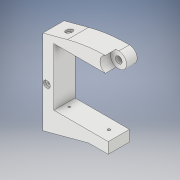
# Autodesk Inventor part: Riser Base
Saved by Autodesk Inventor 2017 SP1 (Build 210196100, 196)
## iProperties
Created: 2017-07-19
Part Number: Riser Base
Material: ABS Plastic
Document SubType Name: Modeling
Designer: zallen
Density: 1.06 g/cm^3
Appearance: CR White
Author: zallen
Autodesk Inventor part; units mm, degrees
ref_plane "YZ Plane" through (0, 0, 0) normal (1, 0, 0) x (0, 1, 0)
ref_plane "XZ Plane" through (0, 0, 0) normal (0, 1, 0) x (-1, 0, 0)
ref_plane "XY Plane" through (0, 0, 0) normal (0, 0, 1) x (1, 0, 0)
sketch "Sketch1" plane through (0, 0, 0) normal (0, 0, 1) x (1, 0, 0)
  line L0 (0, 0) -> (160, 0) construction
  line L1 (160, 0) -> (118.589, -154.5481) construction
  line L2 (0, 0) -> (41.411, -154.5481) construction
  line L3 (41.411, -154.5481) -> (118.589, -154.5481)
  circle A0 centre (235.8871, -103.156) radius 80 construction
  line L4 (160, 0) -> (256.5926, -25.8819)
  line L5 (118.589, -154.5481) -> (215.1815, -180.43)
  arc A1 (215.1815, -180.43) -> (256.5926, -25.8819) centre (235.8871, -103.156) ccw
  circle A2 centre (-75.8871, -103.156) radius 80 construction
  line L6 (0, 0) -> (-96.5926, -25.8819)
  line L7 (41.411, -154.5481) -> (-55.1815, -180.43)
  arc A3 (-96.5926, -25.8819) -> (-55.1815, -180.43) centre (-75.8871, -103.156) ccw
  arc A4 (160, 0) -> (0, 0) centre (80, -304.672) ccw
  dimension "d0" = 160
  dimension "d1" = 160
  dimension "d2" = 160
  dimension "d3" = 75
  dimension "d4" = 75
  dimension "d5" = 160
  dimension "d6" = 100
  dimension "d7" = 160
  dimension "d9" = 100
  dimension "d56" = 315
  constraints: 16 end point, 10 point on circle, 8 tangent, 5 centre point, 2 concentric, 2 parallel, 1 horizontal
  measures "d0" distance of L0.start L0.end
  measures "d1" distance of L0.end L1.end
  measures "d2" distance of L0.start L2.end
  measures "d3" angle of L0 L2
  measures "d4" angle of L0 L1
  measures "d5" diameter of A0
  measures "d6" distance of L0.end L4.end
  measures "d7" diameter of A2
  measures "d9" distance of L0.start L6.end
  measures "d56" radius of A4
extrude "Extrusion1" add sketch "Sketch1" along normal blind 41.5
sketch "Sketch2" plane through (0, 0, 41.5) normal (0, 0, 1) x (1, 0, 0)
  line L0 (-26.5, -133) -> (186.5, -133)
  line L1 (186.5, -133) -> (186.5, -20)
  line L2 (186.5, -20) -> (-26.5, -20)
  line L3 (-26.5, -20) -> (-26.5, -133)
  line L4 (0, 0) -> (-96.5926, -25.8819) projected
  arc A0 (160, 0) -> (0, 0) centre (80, -304.672) ccw projected
  line L5 (0, 0) -> (160, 0)
  point P0 (80, -20)
  point P1 (80, 0)
  dimension "d12" = 213
  dimension "d13" = 113
  dimension "d57" = 20
  constraints: 10 end point, 2 horizontal, 2 midpoint, 2 parallel, 1 perpendicular, 1 vertical alignment
  measures "d12" distance of L2.end L1.end
  measures "d13" distance of L1.end L0.end
  measures "d57" distance between parallel lines of L2 L5
extrude "Extrusion2" cut sketch "Sketch2" against normal through all contours L3 L2 L1 L0
sketch "Sketch3" plane through (0, 0, 41.5) normal (0, 0, 1) x (1, 0, 0)
  line L0 (186.5, -20) -> (186.5, -133) construction
  line L1 (186.5, -133) -> (-26.5, -133) construction
  line L2 (-26.5, -133) -> (-26.5, -20) construction
  line L3 (-26.5, -20) -> (186.5, -20) construction
  line L4 (0, 0) -> (-96.5926, -25.8819) construction
  arc A0 (-96.5926, -25.8819) -> (-55.1815, -180.43) centre (-75.8871, -103.156) ccw construction
  line L5 (-55.1815, -180.43) -> (41.411, -154.5481) construction
  line L6 (41.411, -154.5481) -> (118.589, -154.5481) construction
  line L7 (118.589, -154.5481) -> (215.1815, -180.43) construction
  arc A1 (215.1815, -180.43) -> (256.5926, -25.8819) centre (235.8871, -103.156) ccw construction
  line L8 (256.5926, -25.8819) -> (160, 0) construction
  line L9 (-48.0481, -154.5481) -> (208.0481, -154.5481) construction
  line L10 (208.0481, -154.5481) -> (208.0481, 10.328) construction
  line L11 (-48.0481, 10.328) -> (-48.0481, -154.5481) construction
  line L12 (-48.0481, 10.328) -> (-48.0481, -178.5186)
  line L13 (-55.1815, -180.43) -> (41.411, -154.5481) projected
  line L14 (208.0481, 10.328) -> (208.0481, -178.5186)
  line L15 (118.589, -154.5481) -> (215.1815, -180.43) projected
  line L16 (-48.0481, -178.5186) -> (208.0481, -178.5186)
  line L17 (-48.0481, 10.328) -> (208.0481, 10.328)
  line L18 (-157.6505, -218.8456) -> (317.6505, -218.8456)
  line L19 (317.6505, -218.8456) -> (317.6505, 50.655)
  line L20 (317.6505, 50.655) -> (-157.6505, 50.655)
  line L21 (-157.6505, 50.655) -> (-157.6505, -218.8456)
  arc A2 (160, 0) -> (0, 0) centre (80, -304.672) ccw projected
  point P0 (80, -154.5481)
  point P1 (80, 10.328)
  point P2 (208.0481, -84.0953)
  point P3 (317.6505, -84.0953)
  point P4 (80, 10.328)
  point P5 (80, -218.8456)
  dimension "d22" = 269.5006
  dimension "d23" = 475.3011
  constraints: 22 end point, 7 midpoint, 4 parallel, 2 perpendicular, 2 point on line, 1 horizontal, 1 horizontal alignment, 1 tangent, 1 vertical, 1 vertical alignment, 1 other
  measures "d22" distance between parallel lines of L18 L20
  measures "d23" distance of L18.start L18.end
extrude "Extrusion3" cut sketch "Sketch3" against normal through all
sketch "Sketch5" plane through (0, 0, 41.5) normal (0, 0, 1) x (1, 0, 0)
  line L0 (118.589, -154.5481) -> (208.0481, -178.5186) projected
  line L1 (208.0481, -178.5186) -> (80, -178.5186)
  line L2 (80, -178.5186) -> (80, 10.328)
  line L3 (80, 10.328) -> (208.0481, 10.328)
  line L4 (208.0481, 10.328) -> (208.0481, -178.5186)
  arc A0 (160, 0) -> (0, 0) centre (80, -304.672) ccw projected
  constraints: 8 end point, 2 parallel, 1 horizontal, 1 perpendicular, 1 point on circle
extrude "Extrusion4" cut sketch "Sketch5" against normal through all
sketch "Sketch6" plane through (0, 0, 0) normal (0, 1, 0) x (-1, 0, 0)
  circle A0 centre (17, 20.75) radius 2
  line L0 (26.5, 41.5) -> (26.5, 0) projected
  point P0 (26.5, 20.75)
  dimension "d24" = 4
  dimension "d58" = 9.5
  constraints: 1 centre point, 1 horizontal alignment, 1 midpoint
  measures "d24" diameter of A0
  measures "d58" distance from line of L0 A0.centre
extrude "Extrusion5" cut sketch "Sketch6" along normal through all both and the other way through all
sketch "Sketch7" plane through (0, 0, 0) normal (0, 1, 0) x (-1, 0, 0)
  circle A0 centre (17, 20.75) radius 2 projected
  circle A1 centre (17, 20.75) radius 6.5
  dimension "d59" = 13
  constraints: 1 centre point, 1 coincident
  measures "d59" diameter of A1
extrude "Extrusion6" cut sketch "Sketch7" against normal blind 10
ref_plane "Work Plane1" through (41.411, -174.5481, 0) normal (0, -1, 0) x (1, 0, 0)
sketch "Sketch8" plane through (41.411, -174.5481, 0) normal (0, -1, 0) x (1, 0, 0)
  circle A0 centre (-58.411, 20.75) radius 2 projected
  circle A1 centre (-58.411, 20.75) radius 6.5
  point P0 (-41.411, 0)
  dimension "d32" = 13
  constraints: 1 centre point, 1 coincident
  measures "d32" diameter of A1
extrude "Extrusion7" cut sketch "Sketch8" against normal blind 10
sketch "Sketch11" plane through (41.411, -154.5481, 0) normal (0, -1, 0) x (1, 0, 0)
  line L0 (0, 41.5) -> (38.589, 41.5) projected
  line L1 (0, 0) -> (0, 41.5) projected
  line L2 (0, 0) -> (38.589, 0) projected
  line L3 (38.589, 0) -> (38.589, 41.5) projected
  circle A0 centre (19.2945, 20.75) radius 2.5
  circle A1 centre (19.2945, 20.75) radius 6.5
  point P0 (-41.411, 0)
  point P1 (0, 20.75)
  point P2 (19.2945, 41.5)
  dimension "d73" = 5
  dimension "d74" = 13
  constraints: 2 centre point, 2 midpoint, 1 coincident, 1 horizontal alignment, 1 vertical alignment
  measures "d73" diameter of A0
  measures "d74" diameter of A1
extrude "Extrusion10" cut sketch "Sketch11" against normal blind 10 contours A1
sketch "Sketch12" plane through (-48.0481, -178.5186, 41.5) normal (-1, 0, 0) x (0, 0, 1)
  line L0 (-41.5, 0) -> (-41.5, 165.6442) projected
  line L1 (0, 0) -> (-41.5, 0) projected
  line L2 (0, 165.6442) -> (0, 0) projected
  line L3 (-41.5, 165.6442) -> (0, 165.6442) projected
  line L4 (-5, 5) -> (-36.5, 5)
  line L5 (-36.5, 5) -> (-36.5, 160.6442)
  line L6 (-36.5, 160.6442) -> (-5, 160.6442)
  line L7 (-5, 160.6442) -> (-5, 5)
  point P0 (-41.5, 178.5186)
  dimension "d43" = 5
  constraints: 8 end point, 3 other
  measures "d43" distance between parallel lines of L2 L7
extrude "Extrusion11" cut sketch "Sketch12" against normal blind 15 contours L4 L5 L6 L7
sketch "Sketch13" plane through (0, 0, 41.5) normal (0, 0, 1) x (1, 0, 0)
  circle A0 centre (-40.0481, -95.6966) radius 2.5
  line L0 (-48.0481, -12.8745) -> (-48.0481, -178.5186) projected
  point P0 (0, 0)
  point P1 (-48.0481, -95.6966)
  dimension "d46" = 5
  dimension "d47" = 8
  constraints: 1 centre point, 1 horizontal alignment, 1 midpoint
  measures "d46" diameter of A0
  measures "d47" distance from line of L0 A0.centre
extrude "Extrusion12" cut sketch "Sketch13" against normal through all
sketch "Sketch14" plane through (0, 0, 41.5) normal (0, 0, 1) x (1, 0, 0)
  circle A0 centre (-40.0481, -95.6966) radius 2.5 projected
  circle A1 centre (-40.0481, -95.6966) radius 6.5
  point P0 (0, 0)
  dimension "d50" = 13
  constraints: 1 centre point, 1 coincident
  measures "d50" diameter of A1
extrude "Extrusion13" cut sketch "Sketch14" against normal blind 4
sketch "Sketch15" plane through (0, 0, 0) normal (0, 0, -1) x (-1, 0, 0)
  circle A0 centre (40.0481, -95.6966) radius 2.5 projected
  circle A1 centre (40.0481, -95.6966) radius 2.5 projected
  circle A2 centre (40.0481, -95.6966) radius 6.5
  point P0 (0, 0)
  dimension "d53" = 13
  constraints: 1 centre point, 1 coincident
  measures "d53" diameter of A2
extrude "Extrusion14" cut sketch "Sketch15" against normal blind 4
sketch "Sketch16" plane through (0, 0, 41.5) normal (0, 0, 1) x (1, 0, 0)
  line L0 (80, -20) -> (80, 10.328) construction
  circle A0 centre (80, -4.836) radius 6.5 construction
  circle A1 centre (80, -4.836) radius 15.164 construction
  arc A2 (80, -20) -> (80, 10.328) centre (80, -4.836) ccw
  arc A3 (80, -11.336) -> (80, 1.664) centre (80, -4.836) ccw
  arc A4 (80, 10.328) -> (0, 0) centre (80, -304.672) ccw projected
  line L1 (80, 10.328) -> (80, 1.664)
  line L2 (80, -11.336) -> (80, -20)
  dimension "d62" = 13
  constraints: 6 point on circle, 4 end point, 3 centre point, 2 point on line, 1 coincident, 1 collinear, 1 concentric, 1 midpoint, 1 vertical, 1 vertical alignment, 3 other
  measures "d62" diameter of A0
extrude "Extrusion15" add sketch "Sketch16" against normal blind 41.5
sketch "Sketch17" plane through (0, 0, 41.5) normal (0, 0, 1) x (1, 0, 0)
  arc A0 (80, -11.336) -> (80, 1.664) centre (80, -4.836) ccw construction
  circle A1 centre (80, -4.836) radius 6.5
  point P0 (0, 0)
  constraints: 1 coincident, 1 vertical alignment, 2 other
extrude "Extrusion16" cut sketch "Sketch17" against normal through all
sketch "Sketch19" plane through (0, 0, 41.5) normal (0, 0, 1) x (1, 0, 0)
  circle A0 centre (80, -4.836) radius 6.5 projected
  arc A1 (80, -20) -> (80, 10.328) centre (80, -4.836) ccw projected
  circle A2 centre (80, -4.836) radius 15.164 construction
  circle A3 centre (80, -4.836) radius 16.164
  point P0 (0, 0)
  dimension "d72" = 1
  constraints: 2 centre point, 1 coincident, 1 concentric
  measures "d72" radial gap between concentric circles of A2 A3
extrude "Extrusion18" cut sketch "Sketch19" against normal blind 20.75
sketch "Sketch20" plane through (60.7055, -154.5481, 20.75) normal (0, -1, 0) x (1, 0, 0)
  circle A0 centre (0, 0) radius 2.5 projected
  point P0 (-60.7055, -20.75)
extrude "Extrusion19" cut sketch "Sketch20" against normal blind 50
body "Solid1"
